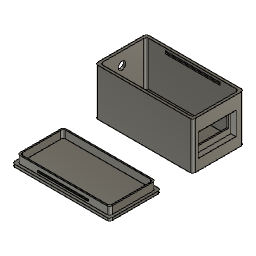
tooth_clock_case (Autodesk Fusion 360 design; units mm, degrees)
Autodesk Fusion 360 part; units mm, degrees
sketch "Sketch1" plane through (0, 0, 0) normal (0, 0, 1) x (1, 0, 0)
  line L0 (0, 0) -> (77, 0)
  line L1 (77, 0) -> (77, 40.5)
  line L2 (77, 40.5) -> (0, 40.5)
  line L3 (0, 40.5) -> (0, 0)
  line L4 (2, 38.5) -> (75, 38.5)
  line L5 (75, 38.5) -> (75, 2)
  line L6 (75, 2) -> (2, 2)
  line L7 (2, 2) -> (2, 38.5)
  circle A0 centre (4, 36.5) radius 2
  circle A1 centre (73, 36.5) radius 2
  circle A2 centre (4, 4) radius 2
  circle A3 centre (73, 4) radius 2
  dimension "d7" = 2
  dimension "d8" = 2
  dimension "d9" = 2
  dimension "d10" = 2
  dimension "d11" = 2
  dimension "d12" = 2
  dimension "d13" = 2
  dimension "d14" = 2
  dimension "d15" = 69
  dimension "d16" = 32.5
  constraint horizontal L0
  constraint vertical L1
  constraint horizontal L2
  constraint vertical L3
  constraint coincident L0.start L3.end
  constraint horizontal L4
  constraint vertical L5
  constraint horizontal L6
  constraint vertical L7
  constraint tangent L4 A0
  constraint tangent L7 A0
  constraint tangent L4 A1
  constraint tangent L5 A1
  constraint tangent L6 A2
  constraint tangent L7 A2
  constraint tangent L5 A3
  constraint tangent L6 A3
  measures "d7" distance of L3 L7
  measures "d8" distance of L2 L4
  measures "d9" distance of L1 L5
  measures "d10" distance of L0 L6
  measures "d11" radius of A0
  measures "d12" radius of A1
  measures "d13" radius of A2
  measures "d14" radius of A3
  measures "d15" distance of A2.centre A3.centre
  measures "d16" distance of A0.centre A2.centre
extrude "Extrude1" add sketch "Sketch1" along normal blind 37 makes body 1
extrude "Extrude2" add sketch "Sketch1" along normal blind 2 separate body contours L4 L7 A0 | L4 L5 L6 L7 A0 A1 A2 A3 | A0 | L4 L5 A1 | A1 | L6 L7 A2 | A2 | A3 | L5 L6 A3 makes body 2
sketch "Sketch4" plane through (0, 0, 2) normal (0, 0, 1) x (-1, 0, 0)
  line L0 (-2, -4) -> (-2, -34.5)
  line L1 (-2, -19.9) -> (-51.84, -19.9)
  line L2 (-51.84, -19.9) -> (-51.84, -21.9)
  line L3 (-51.84, -21.9) -> (-2, -21.9)
  line L4 (-2, -21.9) -> (-2, -19.9)
  line L5 (-2, -2) -> (-75, -2)
  line L6 (-75, -2) -> (-75, -36.5)
  line L7 (-75, -36.5) -> (-2, -36.5)
  line L8 (-2, -36.5) -> (-2, -2)
  line L9 (-2, -2) -> (-75, -2)
  line L10 (-75, -2) -> (-75, -38.5)
  line L11 (-75, -38.5) -> (-2, -38.5)
  line L12 (-2, -38.5) -> (-2, -2)
  line L13 (-77, -40.5) -> (0, -40.5)
  dimension "d56" = 2
  dimension "d139" = 18.6
  constraint horizontal L1
  constraint vertical L2
  constraint horizontal L3
  constraint vertical L4
  constraint coincident L0 L1.start
  measures "d56" distance of L1.start L3.end
  measures "d139" distance of L3 L13
extrude "Extrude7" add sketch "Sketch4" along normal blind 11.6667 contours L0 L1 L2 L3 L4 L8 L12 bodies 1 2
sketch "Sketch6" plane through (75, 0, 0) normal (-1, 0, 0) x (0, -1, 0)
  line L0 (-34.5, 2) -> (-4, 2)
  line L1 (-4, 2) -> (-4, 37)
  line L2 (-4, 37) -> (-34.5, 37)
  line L3 (-34.5, 37) -> (-34.5, 2)
  line L4 (-19.25, 2) -> (-19.25, 17.5)
  line L5 (-32.25, 24.5) -> (-6.25, 24.5)
  line L6 (-6.25, 24.5) -> (-6.25, 10.5)
  line L7 (-6.25, 10.5) -> (-32.25, 10.5)
  line L8 (-32.25, 10.5) -> (-32.25, 24.5)
  line L9 (-32.25, 24.5) -> (-6.25, 10.5) construction
  line L10 (-6.25, 24.5) -> (-32.25, 10.5) construction
  circle A0 centre (-30.75, 26.3) radius 0.75
  circle A1 centre (-7.75, 26.3) radius 0.75
  circle A2 centre (-30.75, 3.3) radius 0.75
  circle A3 centre (-7.75, 3.3) radius 0.75
  line L11 (-30.75, 26.3) -> (-7.75, 26.3)
  line L12 (-19.25, 24.5) -> (-19.25, 26.3)
  line L13 (-38.5, 2) -> (-2, 2)
  line L14 (-2, 2) -> (-2, 37)
  line L15 (-2, 37) -> (-38.5, 37)
  line L16 (-38.5, 37) -> (-38.5, 2)
  point P0 (-19.25, 17.5)
  point P1 (-19.25, 26.3)
  dimension "d61" = 15.5
  dimension "d62" = 26
  dimension "d63" = 14
  dimension "d64" = 1.5
  dimension "d77" = 23
  dimension "d78" = -23
  dimension "d79" = 1.8
  constraint midpoint L0 L4.start
  constraint perpendicular L0 L4
  constraint horizontal L5
  constraint perpendicular L5 L6
  constraint parallel L5 L7
  constraint parallel L6 L8
  constraint coincident L9 P0
  constraint coincident L10 P0
  constraint coincident P0 L4.end
  constraint coincident A0.centre L11.start
  constraint coincident A1.centre L11.end
  constraint midpoint L5 L12.start
  constraint coincident L11 P1
  constraint perpendicular L11 L12
  constraint midpoint L11 P1
  constraint coincident P1 L12.end
  measures "d61" distance of L4.start P0
  measures "d62" distance of L6.end L7.end
  measures "d63" distance of L5.end L6.end
  measures "d64" diameter of A0
  measures "d79" distance of L12.start P1
extrude "Extrude9" cut sketch "Sketch6" against normal up to surface (2 mm away) contours L5 L6 L7 L8 bodies 1
chamfer "Chamfer1" distance 2 angle 45 4 edges at (77, 32.25, 17.5) (77, 19.25, 24.5) (77, 19.25, 10.5) (77, 6.25, 17.5) on bodies 1
sketch "Sketch7" plane through (2, 0, 0) normal (1, 0, 0) x (0, 1, 0)
  line L0 (17.9, 2) -> (17.9, 13.6667)
  line L1 (17.9, 13.6667) -> (19.9, 13.6667)
  line L2 (19.9, 13.6667) -> (19.9, 2)
  line L3 (19.9, 2) -> (34.5, 2)
  line L4 (34.5, 2) -> (34.5, 37)
  line L5 (34.5, 37) -> (4, 37)
  line L6 (4, 37) -> (4, 2)
  circle A0 centre (19.25, 27) radius 3
  line L7 (19.25, 37) -> (19.25, 27)
  line L8 (4, 2) -> (17.9, 2)
  line L9 (19.9, 2) -> (19.9, 13.6667)
  line L10 (19.9, 13.6667) -> (21.9, 13.6667)
  line L11 (21.9, 13.6667) -> (21.9, 2)
  line L12 (21.9, 2) -> (38.5, 2)
  line L13 (38.5, 2) -> (38.5, 37)
  line L14 (38.5, 37) -> (2, 37)
  line L15 (2, 37) -> (2, 2)
  line L16 (2, 2) -> (19.9, 2)
  dimension "d80" = 6
  dimension "d82" = 10
  constraint midpoint L5 L7.start
  constraint coincident A0.centre L7.end
  measures "d80" diameter of A0
  measures "d82" distance of L7.start A0.centre
extrude "Extrude10" cut sketch "Sketch7" against normal blind 2 contours A0 bodies 1
sketch "Sketch8" plane through (0, 38.5, 0) normal (0, -1, 0) x (1, 0, 0)
  line L0 (4, 2) -> (73, 2)
  line L1 (73, 2) -> (73, 37)
  line L2 (73, 37) -> (4, 37)
  line L3 (4, 37) -> (4, 2)
  line L4 (71.8, 2) -> (70.8, 2)
  line L5 (70.8, 2) -> (70.8, 12)
  line L6 (70.8, 12) -> (71.8, 12)
  line L7 (71.8, 12) -> (71.8, 2)
  line L8 (75, 29) -> (75, 2)
  line L9 (75, 37) -> (75, 2)
  line L10 (4, 2) -> (73, 2)
  line L11 (73, 2) -> (73, 37)
  line L12 (73, 37) -> (4, 37)
  line L13 (4, 37) -> (4, 2)
  line L14 (2, 2) -> (75, 2)
  line L15 (75, 2) -> (75, 37)
  line L16 (75, 37) -> (2, 37)
  line L17 (2, 37) -> (2, 2)
  dimension "d86" = 1
  dimension "d88" = 10
  dimension "d98" = 3.2
  constraint horizontal L4
  constraint vertical L5
  constraint horizontal L6
  constraint vertical L7
  constraint coincident L0 L4.start
  measures "d86" distance of L4.start L4.end
  measures "d88" distance of L4.end L5.end
  measures "d98" distance of L7 L9
extrude "Extrude11" add sketch "Sketch8" along normal up to surface (36.5 mm away) contours L0 L4 L5 L6 L7 L10 L14 bodies 1
sketch "Sketch9" plane through (0, 0, 12) normal (0, 0, 1) x (-1, 0, 0)
  line L0 (-71.8, -2) -> (-71.8, -38.5)
  line L1 (-70.8, -38.5) -> (-70.8, -2)
  line L2 (-70.8, -33.25) -> (-71.8, -33.25)
  line L3 (-71.8, -33.25) -> (-71.8, -7.25)
  line L4 (-71.8, -7.25) -> (-70.8, -7.25)
  line L5 (-70.8, -7.25) -> (-70.8, -33.25)
  line L6 (-70.8, -2) -> (-71.8, -2)
  line L7 (-71.8, -38.5) -> (-70.8, -38.5)
  point P0 (-70.8, -20.25)
  point P1 (-70.8, -20.25)
  dimension "d91" = 26
  constraint horizontal L2
  constraint vertical L3
  constraint horizontal L4
  constraint vertical L5
  constraint coincident L0 L3.end
  constraint coincident L1 L2.start
  constraint midpoint L1 P1
  constraint midpoint L5 P1
  constraint coincident P1 P0
  measures "d91" distance of L2.start L4.end
extrude "Extrude12" add sketch "Sketch9" along normal blind 17 contours L0 L1 L4 L6 | L0 L1 L2 L7 bodies 1
fillet "Fillet2" radius 5 2 edges at (71.3, 33.25, 29) (71.3, 7.25, 29) on bodies 1
fillet "Fillet3" radius 2 4 edges at (77, 40.5, 18.5) (0, 40.5, 18.5) (0, 0, 18.5) (77, 0, 18.5) on bodies 1
fillet "Fillet4" radius 2 4 edges at (75, 2, 19.5) (75, 38.5, 19.5) (2, 38.5, 19.5) (2, 2, 19.5) on bodies 1
sketch "Sketch10" plane through (0, 2, 0) normal (0, 1, 0) x (-1, 0, 0)
  line L0 (-4, 2) -> (-4, 37)
  line L1 (-4, 37) -> (-73, 37)
  line L2 (-73, 37) -> (-73, 2)
  line L3 (-73, 2) -> (-71.8, 2)
  line L4 (-71.8, 2) -> (-71.8, 29)
  line L5 (-71.8, 29) -> (-70.8, 29)
  line L6 (-70.8, 29) -> (-70.8, 2)
  line L7 (-70.8, 2) -> (-4, 2)
  line L8 (-60.1667, 35) -> (-16.8333, 35)
  line L9 (-16.8333, 35) -> (-16.8333, 33)
  line L10 (-16.8333, 33) -> (-60.1667, 33)
  line L11 (-60.1667, 33) -> (-60.1667, 35)
  line L12 (-38.5, 37) -> (-38.5, 35)
  point P0 (-38.5, 35)
  dimension "d103" = 43.3333
  dimension "d104" = 2
  constraint horizontal L8
  constraint vertical L9
  constraint horizontal L10
  constraint vertical L11
  constraint midpoint L8 P0
  constraint midpoint L1 L12.start
  constraint coincident L8 P0
  constraint perpendicular L8 L12
  constraint coincident P0 L12.end
  measures "d103" distance of L8.start L8.end
  measures "d104" distance of L8.end L9.end
extrude "Extrude13" cut sketch "Sketch10" against normal blind 1 contours L8 L9 L10 L11 bodies 1
ref_plane "WorkPlane2" through (38.5, 20.25, 19.5) normal (0, -1, 0) x (1, 0, 0)
mirror "Mirror1" about plane through (38.5, 20.25, 19.5) normal (0, -1, 0) of "Extrude13"
sketch "Sketch11" plane through (0, 0, 0) normal (0, 0, 1) x (1, 0, 0)
  line L0 (0, 0) -> (0, -25)
  line L1 (0, -25) -> (77, -25)
  line L2 (77, -25) -> (77, -65.5)
  line L3 (77, -65.5) -> (0, -65.5)
  line L4 (0, -65.5) -> (0, -25)
  line L5 (2.1, -27.1) -> (74.9, -27.1)
  line L6 (74.9, -27.1) -> (74.9, -63.4)
  line L7 (74.9, -63.4) -> (2.1, -63.4)
  line L8 (2.1, -63.4) -> (2.1, -27.1)
  dimension "d109" = 77
  dimension "d110" = 40.5
  dimension "d111" = 2.1
  dimension "d112" = 2.1
  dimension "d113" = 2.1
  dimension "d114" = 2.1
  constraint coincident L0.start origin
  constraint vertical L0
  constraint horizontal L1
  constraint vertical L2
  constraint horizontal L3
  constraint vertical L4
  constraint horizontal L5
  constraint vertical L6
  constraint horizontal L7
  constraint vertical L8
  measures "d109" distance of L0.end L1.end
  measures "d110" distance of L0.end L3.end
  measures "d111" distance of L2 L6
  measures "d112" distance of L1 L5
  measures "d113" distance of L4 L8
  measures "d114" distance of L3 L7
extrude "Extrude14" add sketch "Sketch11" along normal blind 2 separate body contours L1 L2 L3 L4 | L5 L6 L7 L8 makes body 3
extrude "Extrude15" add sketch "Sketch11" along normal blind 8 contours L5 L6 L7 L8 bodies 3
sketch "Sketch12" plane through (0, 0, 8) normal (0, 0, 1) x (-1, 0, 0)
  line L0 (-2.1, 63.4) -> (-74.9, 63.4)
  line L1 (-74.9, 63.4) -> (-74.9, 27.1)
  line L2 (-74.9, 27.1) -> (-2.1, 27.1)
  line L3 (-2.1, 27.1) -> (-2.1, 63.4)
  line L4 (-73.9, 62.4) -> (-3.1, 62.4)
  line L5 (-3.1, 62.4) -> (-3.1, 28.1)
  line L6 (-3.1, 28.1) -> (-73.9, 28.1)
  line L7 (-73.9, 28.1) -> (-73.9, 62.4)
  dimension "d120" = 1
  dimension "d121" = 1
  dimension "d122" = 1
  dimension "d123" = 1
  constraint horizontal L4
  constraint vertical L5
  constraint horizontal L6
  constraint vertical L7
  measures "d120" distance of L3 L5
  measures "d121" distance of L1 L7
  measures "d122" distance of L0 L4
  measures "d123" distance of L2 L6
extrude "Extrude16" cut sketch "Sketch12" against normal blind 6 contours L4 L5 L6 L7 bodies 3
fillet "Fillet5" radius 2 8 edges at (2.1, -63.4, 5) (74.9, -63.4, 5) (73.9, -28.1, 5) (3.1, -28.1, 5) (74.9, -27.1, 5) (3.1, -62.4, 5) (2.1, -27.1, 5) (73.9, -62.4, 5) on bodies 3
fillet "Fillet5" radius 2 4 edges at (77, -25, 1) (77, -65.5, 1) (0, -25, 1) (0, -65.5, 1) on bodies 3
sketch "Sketch13" plane through (0, -63.4, 0) normal (0, -1, 0) x (1, 0, 0)
  line L0 (72.9, 2) -> (72.9, 8)
  line L1 (72.9, 8) -> (4.1, 8)
  line L2 (4.1, 8) -> (4.1, 2)
  line L3 (4.1, 2) -> (72.9, 2)
  line L4 (18.5, 5) -> (58.5, 5)
  line L5 (58.5, 5) -> (58.5, 4.2)
  line L6 (58.5, 4.2) -> (18.5, 4.2)
  line L7 (18.5, 4.2) -> (18.5, 5)
  line L8 (38.5, 2) -> (38.5, 4.2)
  point P0 (38.5, 4.2)
  dimension "d130" = 0.8
  dimension "d131" = 40
  dimension "d135" = 2.2
  constraint horizontal L4
  constraint vertical L5
  constraint horizontal L6
  constraint vertical L7
  constraint midpoint L3 L8.start
  constraint coincident L6 P0
  constraint perpendicular L6 L8
  constraint midpoint L6 P0
  constraint coincident P0 L8.end
  measures "d130" distance of L4.start L6.end
  measures "d131" distance of L4.start L4.end
  measures "d135" distance of L8.start P0
extrude "Extrude17" add sketch "Sketch13" along normal blind 0.7 contours L4 L5 L6 L7 bodies 3
chamfer "Chamfer2" distance 0.5 angle 45 1 edges at (38.5, -64.1, 5) on bodies 3
ref_plane "WorkPlane3" through (38.5, -45.25, 5) normal (0, -1, 0) x (1, 0, 0)
mirror "Mirror2" about plane through (38.5, -45.25, 5) normal (0, -1, 0) of "Extrude17", "Chamfer2"
equation "innerW = 28.5 mm"
equation "innerD = 65 mm"
equation "innerH = 35 mm"
equation "thickness = 2 mm"
equation "socketOuterD = 2 mm"
equation "socketInnerD = 1.5 mm"
equation "d7 = thickness"
equation "d8 = thickness"
equation "d9 = thickness"
equation "d10 = thickness"
equation "d11 = socketOuterD"
equation "d12 = socketOuterD"
equation "d13 = socketOuterD"
equation "d14 = socketOuterD"
equation "d15 = innerD + 2 * socketOuterD"
equation "d16 = innerW + 2 * socketOuterD"
equation "d17 = innerH + thickness"
equation "d19 = thickness"
equation "socketHoleDepth = 3 mm"
equation "boardLift = 2 mm"
equation "usbVerticalOffset = 1 mm"
equation "displayH = 14 mm"
equation "displayW = 26 mm"
equation "d56 = thickness"
equation "d59 = innerH / 3"
equation "d62 = displayW"
equation "d63 = displayH"
equation "d74 = thickness"
equation "d83 = -1 * thickness"
equation "d100 = thickness"
equation "d102 = thickness"
equation "d103 = 2 * innerD / 3"
equation "d111 = thickness + lidClearance"
equation "d112 = thickness + lidClearance"
equation "d113 = thickness + lidClearance"
equation "d114 = thickness + lidClearance"
equation "lidClearance = 0.1 mm"
equation "d116 = thickness"
equation "d118 = 6 mm + thickness"
equation "d127 = thickness"
equation "d129 = thickness"
named bodies: "Tooth clock body", "Tooth clock lid"
